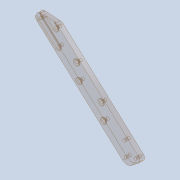
# Autodesk Inventor part: アーム先1
Saved by Autodesk Inventor 2020.4 (Build 244396000, 396)
## iProperties
Created: 2021-05-06
Part Number: アーム先1
Material: ポリカーボネート、スモーク
Document SubType Name: Modeling
Designer: happy
Density: 1.2 g/cm^3
Appearance: ポリカーボネート - スモーク
Mass: 14.7026 g
Surface Area: 70.6344 cm^2
Volume: 12.2522 cm^3
Author: happy
Autodesk Inventor part; units mm, degrees
ref_plane "YZ Plane" through (0, 0, 0) normal (1, 0, 0) x (0, 1, 0)
ref_plane "XZ Plane" through (0, 0, 0) normal (0, 1, 0) x (-1, 0, 0)
ref_plane "XY Plane" through (0, 0, 0) normal (0, 0, 1) x (1, 0, 0)
sketch "スケッチ1" plane through (0, 0, 0) normal (0, 0, 1) x (1, 0, 0)
  circle A0 centre (211.0538, -16.1783) radius 3
  circle A1 centre (195.0769, -15.1842) radius 3
  circle A2 centre (213.5911, -31.9837) radius 3
  line L0 (195.0769, -15.1842) -> (213.5911, -31.9837) construction
  line L1 (185.1065, 0.6143) -> (518.3624, -301.7771) construction
  circle A3 centre (185.1065, 0.6143) radius 8
  line L2 (204.334, -23.584) -> (211.0538, -16.1783) construction
  line L3 (185.1065, 0.6143) -> (181.7466, -3.0885)
  line L4 (181.7466, -3.0885) -> (195.0769, -15.1842)
  line L5 (211.0538, -16.1783) -> (195.0769, -15.1842) construction
  line L6 (213.748, -11.3362) -> (182.759, -9.4081)
  line L7 (186.8707, -14.4897) -> (289.472, -107.5885)
  arc A4 (195.3874, -10.1938) -> (196.9446, -10.5462) centre (195.0769, -15.1842) ccw
  arc A5 (214.4137, -12.4754) -> (211.3643, -11.1879) centre (211.0538, -16.1783) ccw
  line L8 (214.4137, -12.4754) -> (302.9116, -92.7771)
  line L9 (302.9116, -92.7771) -> (289.472, -107.5885) construction
  circle A6 centre (295.8489, -93.1201) radius 3.025
  circle A7 centre (285.4262, -97.1659) radius 3.025
  circle A8 centre (283.9998, -82.3684) radius 3.025
  line L10 (281.7596, -80.3356) -> (285.1195, -76.6328)
  line L11 (285.1195, -76.6328) -> (289.5999, -80.6983)
  line L12 (289.5999, -80.6983) -> (286.24, -84.4011)
  line L13 (286.24, -84.4011) -> (281.7596, -80.3356) construction
  arc A9 (282.4058, -101.1768) -> (291.3448, -101.5663) centre (287.1097, -95.9928) ccw
  line L14 (302.9116, -92.7771) -> (291.3448, -101.5663)
  arc A10 (299.0788, -95.6895) -> (299.3467, -89.5424) centre (296.6588, -92.5047) ccw
  circle A11 centre (295.8489, -93.1201) radius 1.5
  circle A12 centre (285.4262, -97.1659) radius 1.5
  line L15 (213.5911, -31.9837) -> (181.7466, -3.0885) construction
  line L16 (215.607, -29.762) -> (183.7626, -0.8668)
  line L17 (179.7307, -5.3102) -> (211.5751, -34.2054)
  arc A13 (211.5751, -34.2054) -> (215.607, -29.762) centre (213.5911, -31.9837) ccw
  arc A14 (183.7626, -0.8668) -> (179.7307, -5.3102) centre (181.7466, -3.0885) ccw
  line L18 (211.0538, -16.1783) -> (189.2132, 3.6395) construction
  line L19 (209.0378, -18.4) -> (187.1973, 1.4178)
  line L20 (191.2292, 5.8612) -> (213.0697, -13.9566)
  arc A15 (209.0378, -18.4) -> (213.0697, -13.9566) centre (211.0538, -16.1783) ccw
  arc A16 (191.2292, 5.8612) -> (187.1973, 1.4178) centre (189.2132, 3.6395) ccw
  circle A17 centre (195.0769, -15.1842) radius 1.5
  circle A18 centre (211.0538, -16.1783) radius 1.5
  circle A19 centre (213.5911, -31.9837) radius 1.5
  circle A20 centre (283.9998, -82.3684) radius 1.5
  circle A21 centre (233.2708, -36.3377) radius 3.025
  circle A22 centre (235.8081, -52.1431) radius 3.025
  circle A23 centre (259.1907, -59.857) radius 3.025
  circle A24 centre (261.728, -75.6625) radius 3.025
  line L21 (211.0538, -16.1783) -> (283.9998, -82.3684) construction
  line L22 (285.4262, -97.1659) -> (213.5911, -31.9837) construction
  circle A25 centre (233.2708, -36.3377) radius 1.5
  circle A26 centre (235.8081, -52.1431) radius 1.5
  circle A27 centre (259.1907, -59.857) radius 1.5
  circle A28 centre (261.728, -75.6625) radius 1.5
  point P0 (0, 0)
  point P1 (0, 0)
  point P2 (207.6939, -19.8811)
  point P3 (191.717, -18.887)
  point P4 (197.6688, -17.5361)
  point P5 (200.1335, -6.2694)
  point P6 (209.9194, -11.098)
  point P7 (200.3333, -10.5016)
  point P8 (194.1305, -10.2746)
  point P9 (196.0232, -20.0938)
  point P10 (289.5999, -80.6983)
  point P11 (286.24, -84.4011)
  point P12 (190.0986, -14.718)
  dimension "d13" = 6.05
  dimension "d0" = 6
  dimension "d1" = 25
  dimension "d2" = 10
  dimension "d3" = 18
  dimension "d4" = 5
  dimension "d5" = 5
  dimension "d6" = 150
  dimension "d7" = 6.05
  dimension "d8" = 5
  dimension "d9" = 5
  dimension "d10" = 6.05
  dimension "d11" = 5
  dimension "d12" = 10
  dimension "d14" = 5
  dimension "d15" = 16
  dimension "d16" = 4
  dimension "d17" = 7
  dimension "d18" = 4
  dimension "d19" = 3
  dimension "d20" = 3
  dimension "d23" = 3
  dimension "d24" = 3
  dimension "d25" = 3
  dimension "d26" = 3
  dimension "d29" = 30
  dimension "d30" = 30
  dimension "d31" = 35
  dimension "d32" = 35
  dimension "d33" = 3
  dimension "d34" = 3
  dimension "d35" = 3
  dimension "d36" = 3
  constraints: 50 end point, 28 centre point, 16 point on circle, 16 tangent, 13 coincident, 11 point on line, 10 parallel, 5 equal radius, 5 midpoint, 5 perpendicular, 1 collinear, 1 concentric, 6 other
  measures "d0" diameter of A1
  measures "d1" distance of L0.start L0.end
  measures "d2" distance from line of L0 L2.end
  measures "d3" distance of L3.end L0.start
  measures "d4" distance between parallel lines of L6 L5
  measures "d5" distance from line of L7 L0.start
  measures "d6" distance from line of L3.start L9
  measures "d7" diameter of A6
  measures "d8" distance from line of L1 A6.centre
  measures "d9" distance from line of L9 A6.centre
  measures "d10" diameter of A7
  measures "d11" distance from line of A7.centre L1
  measures "d12" distance from line of L9 A7.centre
  measures "d14" distance from line of L1 point (284, -82.368)
  measures "d15" distance of A6.centre point (284, -82.368)
  measures "d16" distance from line of L14 A6.centre
  measures "d17" radius of A9
  measures "d18" radius of A10
  measures "d19" diameter of A11
  measures "d20" diameter of A12
  measures "d23" diameter of A17
  measures "d24" diameter of A18
  measures "d25" diameter of A19
  measures "d26" diameter of A20
  measures "d29" distance of A21.centre L2.end
  measures "d30" distance of A22.centre L0.end
  measures "d31" distance of A23.centre A21.centre
  measures "d32" distance of A22.centre A24.centre
  measures "d33" diameter of A25
  measures "d34" diameter of A26
  measures "d35" diameter of A27
  measures "d36" diameter of A28
extrude "押し出し1" add sketch "スケッチ1" along normal blind 5 contours A0 L20 L6 A5 L8 L10 A8 L12 A10 L14 A9 L7 A4 L17 A2 L16 L19 | L8 L12 A8 L10 | A8 | L17 A4 | A6 | A7
extrude "押し出し2" add sketch "スケッチ1" along normal blind 4 contours A0 | A0 L19 L6 L20 | L16 A1 L4 A4 | L4 A1 L17 A4 | L16 A4 L17 A1 | A1 | L16 A2 L17 A4 | A2 | A21 | A22 | A23 | A24
